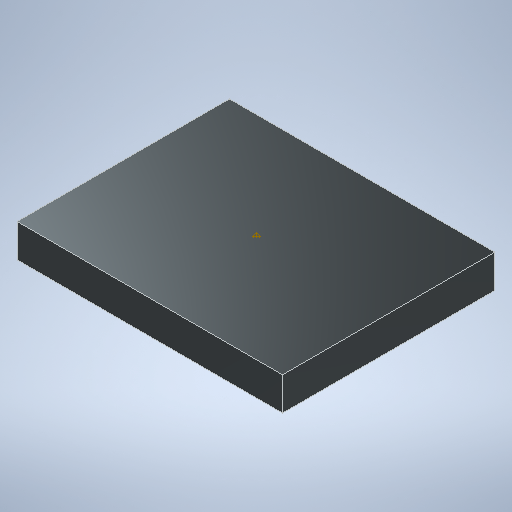
# Autodesk Inventor part: graphite_new
Saved by Autodesk Inventor 2025 (Build 290162000, 162)
## iProperties
Created: 2025-05-20
Part Number: graphite_new
Material: Iron, Ductile
Document SubType Name: Modeling
Designer: warke
Density: 7.15 g/cm^3
Appearance: Iron Gray
Author: warke
Autodesk Inventor part; units mm, degrees
ref_plane "YZ Plane" through (0, 0, 0) normal (1, 0, 0) x (0, 1, 0)
ref_plane "XZ Plane" through (0, 0, 0) normal (0, 1, 0) x (-1, 0, 0)
ref_plane "XY Plane" through (0, 0, 0) normal (0, 0, 1) x (1, 0, 0)
sketch "Sketch1" plane through (0, 0, 0) normal (0, 1, 0) x (-1, 0, 0)
  line L0 (-2, 1.6) -> (2, 1.6)
  line L1 (2, 1.6) -> (2, -1.6)
  line L2 (2, -1.6) -> (-2, -1.6)
  line L3 (-2, -1.6) -> (-2, 1.6)
  line L4 (-2, 1.6) -> (2, -1.6) construction
  line L5 (2, 1.6) -> (-2, -1.6) construction
  point P0 (0, 0)
  dimension "d0" = 4
  dimension "d1" = 3.2
  constraints: 12 end point, 2 midpoint, 2 parallel, 1 horizontal, 1 perpendicular
  measures "d0" distance of L1.end L2.end
  measures "d1" distance of L0.end L1.end
extrude "Extrusion1" add sketch "Sketch1" along normal blind 0.5
body "Solid1"
